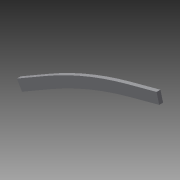
# Autodesk Inventor part: nd-o
Saved by Autodesk Inventor 2015 (Build 190159000, 159)
## iProperties
Created: 2014-07-02
Part Number: nd-o
Material: Generic
Document SubType Name: Modeling
Designer: peter
Density: 1 g/cm^3
Appearance: Default
Author: peter
Autodesk Inventor part; units mm, degrees
ref_plane "YZ Plane" through (0, 0, 0) normal (1, 0, 0) x (0, 1, 0)
ref_plane "XZ Plane" through (0, 0, 0) normal (0, 1, 0) x (-1, 0, 0)
ref_plane "XY Plane" through (0, 0, 0) normal (0, 0, 1) x (1, 0, 0)
sketch "Sketch1" plane through (0, 0, 0) normal (0, 0, 1) x (1, 0, 0)
  line L0 (707.9241, 284.5068) -> (560.717, 245.0627)
  arc A0 (560.717, 245.0627) -> (168.6533, 82.6646) centre (981.4533, -1325.1463) ccw
  line L1 (168.6533, 82.6646) -> (25.4001, -0.0426)
  line L2 (25.4001, -0.0426) -> (0.0001, 43.9515)
  line L3 (0.0001, 43.9515) -> (143.2533, 126.6587)
  arc A1 (547.569, 294.1318) -> (143.2533, 126.6587) centre (981.4533, -1325.1463) ccw
  line L4 (547.569, 294.1318) -> (694.7761, 333.5758)
  line L5 (694.7761, 333.5758) -> (707.9241, 284.5068)
  point P0 (0, 0)
  constraints: 12 end point, 4 point on circle, 2 centre point
extrude "Extrusion1" add sketch "Sketch1" along normal blind 19.05
body "Solid1"
